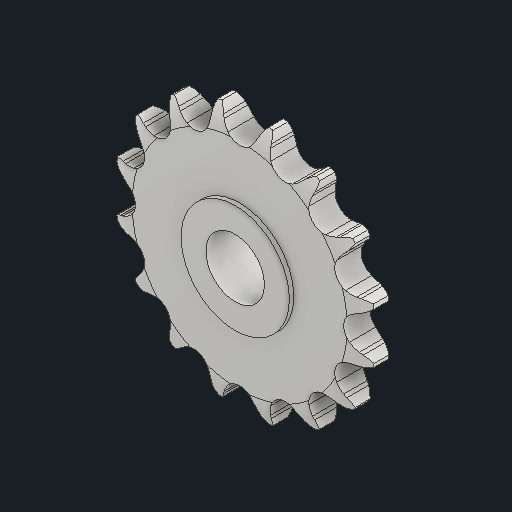
# Autodesk Inventor part: Roller Chain Sprocket1
Saved by Autodesk Inventor 2027 (Build 310192000, 192)
## iProperties
CustomPartVersion: 1
Created: 2026-06-06
Part Number: Roller Chain Sprocket1
Material: Steel
Document SubType Name: Modeling
Designer: W Ahmad
Density: 1 g/cm^3
Appearance: Steel
Author: W Ahmad
Autodesk Inventor part; units mm, degrees
ref_plane "YZ Plane" through (0, 0, 0) normal (1, 0, 0) x (0, 1, 0)
ref_plane "XZ Plane" through (0, 0, 0) normal (0, 1, 0) x (-1, 0, 0)
sketch "Theoretical Tooth Profile" plane through (0, 0, 0) normal (0, 0, 1) x (1, 0, 0)
  circle A0 centre (0, 0) radius 40.6863 construction
  line L0 (0, 0) -> (0, 40.6863) construction
  line L1 (0, 0) -> (15.57, 37.5892) construction
  circle A1 centre (0, 0) radius 44.667
  arc A2 (-4.0113, 37.4668) -> (4.0113, 37.4668) centre (0, 40.6863) ccw
  line L2 (0, 40.6863) -> (15.57, 37.5892) construction
  line L3 (0, 40.6863) -> (6.3389, 45.7738) construction
  line L4 (6.3389, 45.7738) -> (-5.7615, 40.3229) construction
  arc A3 (8.0207, 43.941) -> (6.2399, 41.3848) centre (13.9507, 37.9113) ccw
  arc A4 (-6.2399, 41.3848) -> (-8.0207, 43.941) centre (-13.9507, 37.9113) ccw
  line L5 (-13.9507, 37.9113) -> (-6.2399, 41.3848) construction
  arc A5 (-5.7615, 40.3229) -> (-4.0113, 37.4668) centre (6.3389, 45.7738) ccw
  line L6 (-5.7615, 40.3229) -> (-6.2399, 41.3848)
  arc A6 (4.0113, 37.4668) -> (5.7615, 40.3229) centre (-6.3389, 45.7738) ccw
  line L7 (6.2399, 41.3848) -> (5.7615, 40.3229)
  line L8 (0, 0) -> (8.7141, 43.8087) construction
  point P0 (7.785, 39.1378)
  dimension "d0" = 81.3726
  dimension "d2" = 22.5
  dimension "d3" = 5.1435
  dimension "d10" = 128.75
  dimension "d11" = 14.5
  dimension "d12" = 8.128
  dimension "d13" = 13.2715
  dimension "d14" = 14.224
  dimension "d23" = 4.7625
  constraints: 18 end point, 15 point on circle, 7 centre point, 3 coincident, 3 point on line, 3 symmetric about line, 3 tangent, 1 equal radius, 1 midpoint, 1 parallel, 1 vertical, 1 other
  measures "d0" diameter of A0
  measures "d2" angle of L1 L0
  measures "d3" radius of A2
  measures "d10" angle of L3 L0
  measures "d11" angle of L4 L3
  measures "d12" distance of L2.start L3.end
  measures "d13" distance of L3.end L4.end
  measures "d14" distance of A3.centre L0.end
  measures "d23" distance from line of L8.end L2
sketch "Tooth Profile" plane through (0, 0, 0) normal (0, 0, 1) x (1, 0, 0)
  circle A0 centre (0, 0) radius 44.667 projected
  line L0 (0, 0) -> (0, 40.6863) construction
  line L1 (0, 40.6863) -> (4.7412, 38.6921) construction
  arc A1 (-4.7412, 38.6921) -> (4.7412, 38.6921) centre (0, 40.6863) ccw
  line L2 (-4.7412, 38.6921) -> (0, 40.6863) construction
  arc A2 (-4.7412, 38.6921) -> (-7.8912, 43.9644) centre (-24.9702, 30.1834) ccw
  arc A3 (7.8912, 43.9644) -> (4.7412, 38.6921) centre (24.9702, 30.1834) ccw
  dimension "d44" = 134.375
  dimension "d45" = 5.1435
  dimension "d46" = 21.9456
  constraints: 8 point on circle, 7 end point, 3 centre point, 2 tangent, 1 coincident, 1 equal radius, 1 symmetric about line, 1 vertical
  measures "d44" angle of L1 L2
  measures "d45" radius of A1
  measures "d46" radius of A3
sketch "Section Profile" plane through (0, 0, 0) normal (1, 0, 0) x (0, 1, 0)
  line L0 (44.667, 0) -> (-44.667, 0) projected
  line L1 (30.951, 4.5053) -> (-30.951, 4.5053)
  line L2 (-30.951, 4.5053) -> (-30.951, -4.5053)
  line L3 (-30.951, -4.5053) -> (30.951, -4.5053)
  line L4 (30.951, -4.5053) -> (30.951, 4.5053)
  line L5 (30.951, 4.5053) -> (44.667, 4.5053) construction
  line L6 (44.667, 4.5053) -> (44.667, -4.5053) construction
  line L7 (44.667, -4.5053) -> (30.951, -4.5053) construction
  line L8 (30.951, -4.5053) -> (30.951, 4.5053)
  arc A0 (44.667, 2.521) -> (36.7275, 4.5053) centre (36.7275, -12.3698) ccw
  arc A1 (36.7275, -4.5053) -> (44.667, -2.521) centre (36.7275, 12.3698) ccw
  line L9 (36.7275, 4.5053) -> (0, 4.5053)
  line L10 (0, 4.5053) -> (0, -4.5053)
  line L11 (0, -4.5053) -> (36.7275, -4.5053)
  line L12 (0, 4.5053) -> (0, -4.5053)
  line L13 (44.667, 2.521) -> (44.667, -2.521)
  point P0 (0, 0)
  point P1 (0, 0)
  dimension "d30" = 9.0107
  dimension "d31" = 61.902
  dimension "d32" = 9.0107
  dimension "d33" = 1.9844
  dimension "d34" = 16.8751
  dimension "d43" = 4.5053
  constraints: 26 end point, 7 midpoint, 5 perpendicular, 4 parallel, 4 point on circle, 3 point on line, 3 symmetric about line, 2 centre point, 2 horizontal, 2 tangent, 1 collinear, 1 other
  measures "d30" distance between parallel lines of L7 L5
  measures "d31" distance between parallel lines of L2 L4
  measures "d32" distance between parallel lines of L3 L1
  measures "d33" distance from line of L13.start L5
  measures "d34" radius of A0
  measures "d43" distance between parallel lines of L3 L0
revolve "Shroud" add sketch "Section Profile" angle 360 about axis through (0, 0, 4.5053) along (0, 0, -1) contours L10 L3 L2 L0 | L0 L2 L1 L10
revolve "Strand" add sketch "Section Profile" angle 360 about axis through (0, 0, 4.5053) along (0, 0, -1) contours L13 A1 L11 L4 L0 | L0 L4 L9 A0 L13 | L4 L3 L10 L0 | L0 L10 L1 L4
fillet "Fillet2" [suppressed]
pattern_of_one "Strand Pattern"
extrude "Theoretical Tooth" cut sketch "Theoretical Tooth Profile" along normal through all both and the other way through all contours A3 L7 A6 A2 A5 L6 A4 A1 picked at (0, 41.5717)
extrude "Tooth" [suppressed]
pattern_circular "Tooth Pattern" count 16 over 360 about axis through (0, 0, -10) along (0, 0, 1) of "Theoretical Tooth"
ref_plane "Timing Plane" through (0, 40.6863, 0) normal (1, 0, 0) x (0, 1, 0)
sketch "Sketch4" plane through (0, 40.6863, 4.5053) normal (0, 0, 1) x (1, 0, 0)
  circle A0 centre (0, -40.6863) radius 10
  dimension "d53" = 20
  constraints: 1 centre point, 1 coincident
  measures "d53" diameter of A0
extrude "Extrusion4" cut sketch "Sketch4" against normal blind 25.4
sketch "Sketch5" plane through (0, 40.6863, 4.5053) normal (0, 0, 1) x (1, 0, 0)
  circle A0 centre (0, -40.6863) radius 10 projected
  circle A1 centre (0, -40.6863) radius 18.5
  dimension "d56" = 37
  constraints: 1 centre point, 1 coincident
  measures "d56" diameter of A1
extrude "Extrusion5" add sketch "Sketch5" along normal blind 1.524 and the other way blind 12.7
equation "\"d3\" = 0.5 * da_Dr + da_SC"
equation "\"d12\" = 0.8 * da_Dr"
equation "\"d13\" = 1.3 * da_Dr + da_SC"
equation "\"d14\" = 1.4 * da_Dr"
equation "\"d23\" = da_Ha"
equation "\"d44\" = da_Alfa"
equation "\"d45\" = da_Ri"
equation "\"d46\" = da_Re"
equation "\"d30\" = da_Bf"
equation "\"d31\" = da_Ds"
equation "\"d32\" = da_Bs"
equation "\"d33\" = da_Ba"
equation "\"d34\" = da_Rx"
equation "\"d51\" = da_Ra"
equation "\"d40\" = da_pt"
equation "\"form_type\" = 0"
equation "\"da_p\" = 15.875"
equation "\"da_Dr\" = 10.16"
equation "\"da_SC\" = 0.0635"
equation "\"da_Ha\" = 4.7625"
equation "\"da_pt\" = 18.1102"
equation "\"da_Bf\" = 9.01065"
equation "\"da_Ba\" = 1.98438"
equation "\"da_Rx\" = 16.87513"
equation "\"da_Ra\" = 0.635"
equation "\"da_Bs\" = 9.01065"
equation "\"da_Ds\" = 61.90201"
equation "\"da_Re\" = 21.9456"
equation "\"da_Ri\" = 5.1435"
equation "\"da_Alfa\" = 134.375deg"
body "Solid1"
